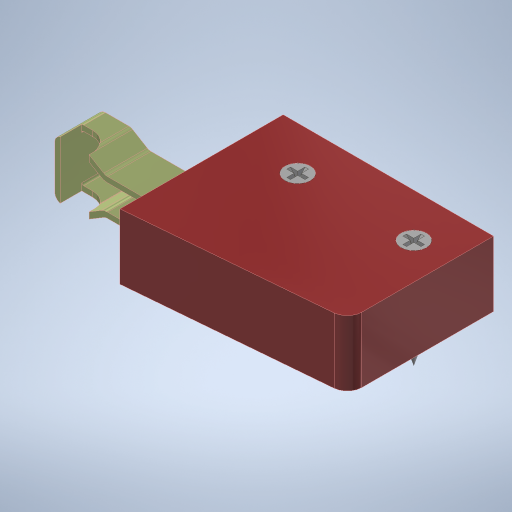
# Autodesk Inventor part: Adjustable universal mounting mechanism T615 Right
Saved by Autodesk Inventor 2024 (Build 280153000, 153)
## iProperties
Category: Wall hanging hardware
Created: 2007-06-13
Part Number: Adjustable universal mounting mechanism T615 Right
Description: Universal adjustable mounting mechanism
Document SubType Name: Modeling
Designer: G.K.
Mass: 44.7999 g
Surface Area: 106.565 cm^2
Volume: 44.7999 cm^3
Density: 1 g/cm^3
Material: Generic
Appearance: Glazed - Firebrick
Authority: Design By CELI APS
Perskaiciuoti: 1
Mase: 0.04479993
Author: G.K.
Title: Universal adjustable mounting mechanism
Subject: Wall hanging hardware
Keywords: Wall hanging hardware, T615, T-600
Comments: Wall hanging hardware, T615, T-600, Wall hanging hardware
Revision Number: 1
Autodesk Inventor part; units mm, degrees
ref_plane "YZ Plane" through (0, 0, 0) normal (1, 0, 0) x (0, 1, 0)
sketch "Sketch1" plane through (0, 0, 0) normal (0, 0, 1) x (1, 0, 0)
  line L0 (0, 0) -> (58, 0)
  line L1 (58, 0) -> (58, -40)
  line L2 (58, -40) -> (0, -45)
  line L3 (0, -45) -> (0, 0)
  dimension "d0" = 45
  dimension "d1" = 58
  dimension "d2" = 40
  constraints: 8 end point, 1 horizontal, 1 parallel, 1 perpendicular
  measures "d0" distance of L2.end L0.start
  measures "d1" distance of L0.start L0.end
  measures "d2" distance of L0.end L1.end
extrude "Extrusion1" add sketch "Sketch1" along normal mid plane 18
ref_plane "Work Plane1" through (0, -23, -9) normal (0, 1, 0) x (1, 0, 0)
sketch "Sketch2" plane through (0, -23, -9) normal (0, 1, 0) x (1, 0, 0)
  line L0 (0, -4) -> (-14, -4)
  line L1 (-14, -4) -> (-14, -14)
  line L2 (-14, -14) -> (0, -14)
  line L3 (0, -14) -> (0, -4)
  line L4 (-19, -1) -> (-28, -1)
  line L5 (-28, -1) -> (-28, -17)
  line L6 (-28, -17) -> (-19, -17)
  line L7 (-19, -17) -> (-19, -1)
  line L8 (-14, -4) -> (-19, -1)
  line L9 (-14, -14) -> (-19, -17)
  line L10 (0, 0) -> (0, -18) projected
  point P0 (0, -9)
  point P1 (0, -9)
  point P2 (-28, -9)
  point P3 (0, -9)
  dimension "d181" = 90
  dimension "d6" = 14
  dimension "d8" = 16
  dimension "d9" = 10
  dimension "d10" = 9
  dimension "d40" = 5
  constraints: 20 end point, 4 midpoint, 4 parallel, 2 horizontal, 2 perpendicular, 1 horizontal alignment
  measures "d6" distance of L0.start L0.end
  measures "d8" distance of L4.end L5.end
  measures "d9" distance between parallel lines of L2 L0
  measures "d10" distance of L4.start L4.end
  measures "d40" horizontal distance of L1.end L6.end
extrude "Extrusion2" add sketch "Sketch2" against normal blind 12
fillet "Fillet1" radius 2 6 edges at (-28, -29, -8) (-28, -29, 8) (-19, -29, -8) (-14, -29, -5) (-14, -29, 5) (-19, -29, 8)
sketch "Sketch5" plane through (0, -23, -9) normal (0, 1, 0) x (1, 0, 0)
  arc A0 (-19.554, -17) -> (-18.525, -16.715) centre (-19.554, -15) ccw projected
  line L0 (-18.525, -16.715) -> (-14.475, -14.285) projected
  arc A1 (-13.446, -14) -> (-14.475, -14.285) centre (-13.446, -16) ccw projected
  line L1 (-13.446, -14) -> (0, -14) projected
  line L2 (0, -4) -> (0, -14) projected
  line L3 (0, -4) -> (-13.446, -4) projected
  arc A2 (-14.475, -3.715) -> (-13.446, -4) centre (-13.446, -2) ccw projected
  line L4 (-14.475, -3.715) -> (-18.525, -1.285) projected
  arc A3 (-18.525, -1.285) -> (-19.554, -1) centre (-19.554, -3) ccw projected
  line L5 (-19.554, -1) -> (-26, -1) projected
  arc A4 (-26, -1) -> (-28, -3) centre (-26, -3) ccw projected
  line L6 (-28, -3) -> (-28, -15) projected
  arc A5 (-28, -15) -> (-26, -17) centre (-26, -15) ccw projected
  line L7 (-26, -17) -> (-19.554, -17) projected
  line L8 (-26, -2.5) -> (-19.554, -2.5)
  arc A6 (-19.2967, -2.5713) -> (-19.554, -2.5) centre (-19.554, -3) ccw
  line L9 (-19.2967, -2.5713) -> (-15.2468, -5.0012)
  arc A7 (-15.2468, -5.0012) -> (-13.446, -5.5) centre (-13.446, -2) ccw
  line L10 (-13.446, -5.5) -> (-1.5, -5.5)
  line L11 (-1.5, -5.5) -> (-1.5, -12.5)
  line L12 (-1.5, -12.5) -> (-13.446, -12.5)
  arc A8 (-13.446, -12.5) -> (-15.2468, -12.9988) centre (-13.446, -16) ccw
  line L13 (-15.2468, -12.9988) -> (-19.2967, -15.4287)
  arc A9 (-19.554, -15.5) -> (-19.2967, -15.4287) centre (-19.554, -15) ccw
  line L14 (-19.554, -15.5) -> (-26, -15.5)
  arc A10 (-26.5, -15) -> (-26, -15.5) centre (-26, -15) ccw
  line L15 (-26.5, -15) -> (-26.5, -3)
  arc A11 (-26, -2.5) -> (-26.5, -3) centre (-26, -3) ccw
  point P0 (0, -9)
  dimension "d18" = 1.5
  constraints: 16 end point, 12 point on circle, 6 centre point, 13 other
  measures "d18" distance between parallel lines of L6 L15
extrude "Extrusion4" cut sketch "Sketch5" against normal through all contours L8 A6 L9 A7 L10 L11 L12 A8 L13 A9 L14 A10 L15 A11
sketch "Sketch4" plane through (0, 0, 0) normal (0, 0, 1) x (1, 0, 0)
  line L0 (-26.5, -23) -> (-26.5, -35) projected
  line L1 (-26.5, -29) -> (-23.5, -29)
  arc A0 (-18.5, -34) -> (-23.5, -29) centre (-23.5, -34) ccw
  line L2 (-18.5, -34) -> (-18.5, -35)
  line L3 (-18.5, -35) -> (-26.5, -35)
  line L4 (-26.5, -35) -> (-26.5, -29)
  line L5 (-26, -23) -> (-19.554, -23) projected
  point P0 (0, 0)
  dimension "d21" = 6
  dimension "d22" = 8
  dimension "d23" = 5
  constraints: 8 end point, 2 perpendicular, 2 point on circle, 2 tangent, 1 centre point, 1 collinear, 1 midpoint, 1 parallel
  measures "d21" distance between parallel lines of L5 L1
  measures "d22" distance of L2.end L0.end
  measures "d23" radius of A0
extrude "Extrusion5" cut sketch "Sketch4" along normal through all both and the other way through all
sketch "Sketch6" plane through (0, 0, 9) normal (0, 0, 1) x (1, 0, 0)
  line L0 (0, 0) -> (58, 0) projected
  line L1 (0, -45) -> (0, 0) projected
  line L2 (16, -12) -> (48, -12)
  dimension "d26" = 12
  dimension "d27" = 32
  dimension "d28" = 16
  constraints: 2 end point, 1 perpendicular
  measures "d26" distance between parallel lines of L0 L2
  measures "d27" distance of L2.end L2.start
  measures "d28" distance from line of L1 L2.start
hole "Hole1" at (16, -12, 9) at (48, -12, 9) direction (0, 0, -1) diameter 5 end through all countersink diameter 7 countersink angle 90
chamfer "Chamfer1" distance 1.5 angle 45 2 edges at (16, -9.5, -9) (48, -9.5, -9)
fillet "Fillet2" radius 4 1 edges at (58, -40, 0)
ref_plane "Work Plane2" through (16, -12, -89.7168) normal (-1, 0, 0) x (0, 0, 1)
sketch "Sketch7" plane through (16, -12, -89.7168) normal (-1, 0, 0) x (0, 0, 1)
  line L0 (98.7168, 3.5) -> (98.7168, -3.5) projected
  line L1 (98.7168, -4.2) -> (98.7168, 0.7) construction
  line L2 (102.1168, 0) -> (68.7168, 0)
  line L3 (98.7168, 0) -> (98.7168, -3.5)
  line L4 (98.7168, -3.5) -> (98.2168, -3.5)
  line L5 (98.2168, -3.5) -> (96.4668, -1.75)
  line L6 (96.4668, -1.75) -> (74.4408, -1.75)
  line L7 (74.4408, -1.75) -> (68.7168, 0)
  point P0 (89.7168, 12)
  point P1 (74.4408, 0)
  dimension "d42" = 3.5
  dimension "d43" = 7
  dimension "d44" = 0.5
  dimension "d45" = 45
  dimension "d46" = 30
  dimension "d47" = 17
  dimension "d48" = 22.026
  constraints: 15 end point, 3 perpendicular, 1 collinear, 1 midpoint, 1 parallel, 1 point on line
  measures "d42" diameter of L6 L2
  measures "d43" diameter of L4 L2
  measures "d44" distance from line of L4.end L3
  measures "d45" angle of L5 L3
  measures "d46" distance from line of L2.end L3
  measures "d47" angle of L7 L2
  measures "d48" distance of L5.end L6.end
revolve "Revolution1" add sketch "Sketch7" angle 360 about axis through (16, -12, 12.4) along (0, 0, -1) separate body
sketch "Sketch8" plane through (16, -12, -89.7168) normal (-1, 0, 0) x (0, 0, 1)
  line L0 (98.7168, 3.5) -> (98.7168, -3.5) projected
  line L1 (96.5568, 0) -> (99.0768, 0)
  line L2 (96.9168, 0) -> (96.9168, 0.9896)
  line L3 (96.9168, 0.9896) -> (98.7168, 2.5)
  line L4 (98.7168, 2.5) -> (98.7168, 0)
  line L5 (98.7168, 3.5) -> (98.7168, -3.5)
  point P0 (89.7168, 12)
  dimension "d50" = 40
  dimension "d51" = 1.8
  dimension "d52" = 2.5
  constraints: 10 end point, 2 perpendicular, 2 point on line, 1 collinear, 1 midpoint
  measures "d50" angle of L3 L1
  measures "d51" distance between parallel lines of L2 L4
  measures "d52" distance from line of L1 L3.end
extrude "Extrusion6" cut sketch "Sketch8" along normal mid plane 1 bodies 2
pattern_circular "Circular Pattern1" count 4 over 360 about axis through (16, -12, -4.263) along (0, 0, -1) of "Extrusion6" bodies 2
thread "Thread1" size "M4x0.7" class "6g" standard "ANSI Metric M Profile" full length
pattern_linear "Rectangular Pattern1" count 2 spacing 32 along (1, 0, 0) bodies 2
sketch "Sketch9" plane through (16, -12, -89.7168) normal (-1, 0, 0) x (0, 0, 1)
  line L0 (80.7168, -3.5) -> (80.7168, 3.5)
  line L1 (80.7168, 4.2) -> (80.7168, -0.7) construction
  line L2 (77.3168, 0) -> (110.7168, 0)
  line L3 (80.7168, 0) -> (80.7168, 3.5)
  line L4 (80.7168, 3.5) -> (81.2168, 3.5)
  line L5 (81.2168, 3.5) -> (82.9668, 1.75)
  line L6 (82.9668, 1.75) -> (104.9928, 1.75)
  line L7 (104.9928, 1.75) -> (110.7168, 0)
  line L8 (80.7168, 4) -> (80.7168, -4) projected
  point P0 (89.7168, 12)
  point P1 (89.7168, 12)
  point P2 (104.9928, 0)
  point P3 (80.7168, 0)
  dimension "d64" = 3.5
  dimension "d65" = 7
  dimension "d66" = 0.5
  dimension "d67" = 45
  dimension "d68" = 30
  dimension "d69" = 17
  dimension "d70" = 22.026
  constraints: 17 end point, 3 perpendicular, 2 midpoint, 1 collinear, 1 parallel, 1 point on line
  measures "d64" diameter of L6 L2
  measures "d65" diameter of L4 L2
  measures "d66" distance from line of L4.end L3
  measures "d67" angle of L5 L3
  measures "d68" distance from line of L2.end L3
  measures "d69" angle of L7 L2
  measures "d70" distance of L5.end L6.end
revolve "Revolution2" [suppressed]
sketch "Sketch10" plane through (16, -12, -89.7168) normal (-1, 0, 0) x (0, 0, 1)
  line L0 (82.8768, 0) -> (80.3568, 0)
  line L1 (82.5168, 0) -> (82.5168, -0.9896)
  line L2 (82.5168, -0.9896) -> (80.7168, -2.5)
  line L3 (80.7168, -2.5) -> (80.7168, 0)
  line L4 (80.7168, -3.5) -> (80.7168, 3.5) projected
  point P0 (89.7168, 12)
  point P1 (80.7168, -3.5)
  point P2 (80.7168, 0)
  point P3 (80.7168, -3.5)
  dimension "d72" = 40
  dimension "d73" = 1.8
  dimension "d74" = 2.5
  constraints: 8 end point, 2 perpendicular, 2 point on line
  measures "d72" angle of L2 L0
  measures "d73" distance between parallel lines of L1 L3
  measures "d74" distance from line of L0 L2.end
extrude "Extrusion7" [suppressed]
pattern_circular "Circular Pattern2" [suppressed]
thread "Thread2" size "M4x0.7" class "6g" standard "ANSI Metric M Profile" full length
pattern_linear "Rectangular Pattern2" [suppressed]
sketch "Sketch11" plane through (0, 0, 0) normal (0, 0, 1) x (1, 0, 0)
  line L0 (-30.5, -54) -> (-30.5, -41)
  arc A0 (-28.5, -39) -> (-30.5, -41) centre (-28.5, -41) ccw
  arc A1 (-28.5, -39) -> (-24.5, -35) centre (-28.5, -35) ccw
  line L1 (-24.5, -35) -> (-24.5, -27)
  line L2 (-24.5, -27) -> (-26.5, -27)
  line L3 (-26.5, -27) -> (-26.5, -35)
  arc A2 (-28.5, -37) -> (-26.5, -35) centre (-28.5, -35) ccw
  arc A3 (-28.5, -37) -> (-32.5, -41) centre (-28.5, -41) ccw
  line L4 (-32.5, -41) -> (-32.5, -54)
  arc A4 (-32.5, -54) -> (-28.5, -58) centre (-28.5, -54) ccw
  line L5 (-28.5, -58) -> (-26.5, -58)
  line L6 (-26.5, -58) -> (-26.5, -56)
  line L7 (-26.5, -56) -> (-28.5, -56)
  arc A5 (-30.5, -54) -> (-28.5, -56) centre (-28.5, -54) ccw
  line L8 (-28, -23) -> (-28, -35) projected
  line L9 (-26, -23) -> (-19.554, -23) projected
  point P0 (0, 0)
  point P1 (-32.5, -37)
  point P2 (-26.5, -27)
  dimension "d86" = 1.5
  dimension "d87" = 4
  constraints: 16 end point, 12 point on circle, 6 centre point
  measures "d86" distance from line of point (-26.5, -27) L8
  measures "d87" distance from line of point (-26.5, -27) L9
extrude "Extrusion8" [suppressed]
sketch "Sketch12" plane through (-24.5, -35, 9) normal (1, 0, 0) x (0, 0, -1)
  line L0 (0, 8) -> (125, 8) projected
  line L1 (125, 8) -> (125, 0) projected
  line L2 (3, 8) -> (122, 8)
  line L3 (122, 8) -> (122, 6)
  line L4 (122, 6) -> (3, 6)
  line L5 (3, 6) -> (3, 8)
  line L6 (0, -23) -> (125, -23) projected
  line L7 (122, 8) -> (120, 6)
  line L8 (3, 8) -> (5, 6)
  point P0 (9, 35)
  point P1 (62.5, 8)
  point P2 (62.5, -23)
  point P3 (62.5, 6)
  dimension "d92" = 2
  dimension "d93" = 3
  dimension "d94" = 2
  dimension "d95" = 2
  constraints: 12 end point, 3 midpoint, 3 point on line, 2 parallel, 2 perpendicular, 2 vertical alignment, 1 horizontal
  measures "d92" distance between parallel lines of L0 L4
  measures "d93" distance between parallel lines of L3 L1
  measures "d94" distance of L7.end L3.end
  measures "d95" distance of L8.end L4.end
extrude "Extrusion9" [suppressed]
sketch "Sketch14" plane through (-30.5, -54, 9) normal (1, 0, 0) x (0, 0, -1)
  line L0 (0, 0) -> (0, 13) projected
  line L1 (125, 13) -> (125, 0) projected
  line L2 (62.5, -3.9613) -> (62.5, 48.6353) construction
  line L3 (0, -4) -> (125, -4) projected
  line L4 (0, 13) -> (0, 0)
  line L5 (49.5, 10.5) -> (39.5, 10.5)
  line L6 (39.5, 2.5) -> (49.5, 2.5)
  arc A0 (39.5, 10.5) -> (39.5, 2.5) centre (39.5, 6.5) ccw
  arc A1 (49.5, 2.5) -> (49.5, 10.5) centre (49.5, 6.5) ccw
  line L7 (35.5, 10.5) -> (53.5, 10.5) construction
  line L8 (53.5, 10.5) -> (53.5, 2.5) construction
  line L9 (53.5, 2.5) -> (35.5, 2.5) construction
  line L10 (35.5, 2.5) -> (35.5, 10.5) construction
  line L11 (62.5, -17.1) -> (62.5, 26.3) construction
  circle A2 centre (28.5, 6.5) radius 3
  line L12 (28.5, 6.5) -> (28.5, 32.5416) construction
  line L13 (21.5, 2.5) -> (21.5, 10.5) construction
  arc A3 (17.5, 2.5) -> (17.5, 10.5) centre (17.5, 6.5) ccw
  line L14 (7.5, 10.5) -> (17.5, 10.5)
  line L15 (3.5, 10.5) -> (3.5, 2.5) construction
  line L16 (21.5, 10.5) -> (3.5, 10.5) construction
  line L17 (3.5, 2.5) -> (21.5, 2.5) construction
  arc A4 (7.5, 10.5) -> (7.5, 2.5) centre (7.5, 6.5) ccw
  line L18 (17.5, 2.5) -> (7.5, 2.5)
  line L19 (71.5, 10.5) -> (71.5, 2.5) construction
  arc A5 (75.5, 10.5) -> (75.5, 2.5) centre (75.5, 6.5) ccw
  line L20 (75.5, 10.5) -> (85.5, 10.5)
  line L21 (85.5, 2.5) -> (75.5, 2.5)
  line L22 (89.5, 10.5) -> (71.5, 10.5) construction
  line L23 (71.5, 2.5) -> (89.5, 2.5) construction
  arc A6 (85.5, 2.5) -> (85.5, 10.5) centre (85.5, 6.5) ccw
  line L24 (89.5, 2.5) -> (89.5, 10.5) construction
  circle A7 centre (96.5, 6.5) radius 3
  line L25 (107.5, 2.5) -> (117.5, 2.5)
  line L26 (117.5, 10.5) -> (107.5, 10.5)
  line L27 (121.5, 2.5) -> (103.5, 2.5) construction
  arc A8 (117.5, 2.5) -> (117.5, 10.5) centre (117.5, 6.5) ccw
  line L28 (103.5, 10.5) -> (121.5, 10.5) construction
  line L29 (103.5, 2.5) -> (103.5, 10.5) construction
  arc A9 (107.5, 10.5) -> (107.5, 2.5) centre (107.5, 6.5) ccw
  line L30 (121.5, 10.5) -> (121.5, 2.5) construction
  point P0 (9, 54)
  point P1 (117.5, 6.5)
  point P2 (62.5, -4)
  point P3 (0, 6.5)
  dimension "d105" = 10.5
  dimension "d106" = 7.5
  dimension "d107" = 18
  dimension "d108" = 8
  dimension "d109" = 18
  dimension "d110" = 6
  dimension "d111" = 7
  dimension "d112" = 7.5
  dimension "d113" = 10.5
  constraints: 56 end point, 32 symmetric about line, 16 point on circle, 10 centre point, 6 tangent, 5 parallel, 2 collinear, 2 horizontal, 2 horizontal alignment, 1 midpoint, 1 perpendicular, 7 other
  measures "d105" distance from line of point (117.5, 6.5) L3
  measures "d106" distance from line of L1 point (117.5, 6.5)
  measures "d107" distance of L7.start L8.start
  measures "d108" distance of L9.end L7.start
  measures "d109" diameter of L8 L11
  measures "d110" diameter of A2
  measures "d111" distance from line of L10 L12.start
  measures "d112" distance from line of point (7.5, 6.5) L0
  measures "d113" distance from line of point (7.5, 6.5) L3
extrude "Extrusion10" [suppressed]
ref_plane "Work Plane4" through (-32.5, -47.5, -19.5) normal (0, 0, -1) x (1, 0, 0)
revolve "Revolution3" [suppressed]
sketch "Sketch16" plane through (-32.5, -47.5, -19.5) normal (0, 0, -1) x (1, 0, 0)
  line L0 (2, 5) -> (2, -5) projected
  line L1 (-0.16, 0) -> (2.36, 0)
  line L2 (0.2, 0) -> (0.2, 2.4896)
  line L3 (0.2, 2.4896) -> (2, 4)
  line L4 (2, 4) -> (2, 0)
  line L5 (2, 5) -> (2, -5)
  point P0 (32.5, -47.5)
  dimension "d125" = 40
  dimension "d126" = 1.8
  dimension "d127" = 4
  constraints: 10 end point, 2 perpendicular, 2 point on line, 1 collinear, 1 midpoint
  measures "d125" angle of L3 L1
  measures "d126" distance between parallel lines of L2 L4
  measures "d127" distance from line of L1 L3.end
extrude "Extrusion11" [suppressed]
pattern_circular "Circular Pattern3" [suppressed]
thread "Thread3" size "M5x0.8" class "6g" standard "ANSI Metric M Profile" length 35
pattern_linear "Rectangular Pattern3" [suppressed]
extrude "Extrusion12" [suppressed]
sketch "Sketch17" plane through (-24.5, -35, 116) normal (1, 0, 0) x (0, 0, -1)
  line L0 (0, 8) -> (125, 8) projected
  line L1 (0, 0) -> (0, 8) projected
  line L2 (125, 8) -> (125, 0) projected
  line L3 (3, 8) -> (122, 8)
  line L4 (122, 8) -> (122, 6)
  line L5 (122, 6) -> (3, 6)
  line L6 (3, 6) -> (3, 8)
  line L7 (122, 8) -> (120, 6)
  line L8 (3, 8) -> (5, 6)
  point P0 (116, 35)
  dimension "d143" = 3
  dimension "d144" = 2
  dimension "d145" = 2
  dimension "d146" = 2
  dimension "d147" = 3
  constraints: 12 end point, 3 point on line, 2 parallel, 2 perpendicular, 1 horizontal
  measures "d143" distance between parallel lines of L4 L2
  measures "d144" distance between parallel lines of L0 L5
  measures "d145" distance from line of L8.end L6
  measures "d146" distance of L4.end L7.end
  measures "d147" distance from line of L5.end L1
extrude "Extrusion13" [suppressed]
sketch "Sketch18" plane through (-30.5, -54, 116) normal (1, 0, 0) x (0, 0, -1)
  line L0 (0, 0) -> (0, 13) projected
  line L1 (0, -4) -> (125, -4) projected
  line L2 (0, 13) -> (0, 0)
  line L3 (49.5, 10.5) -> (39.5, 10.5)
  line L4 (39.5, 2.5) -> (49.5, 2.5)
  arc A0 (39.5, 10.5) -> (39.5, 2.5) centre (39.5, 6.5) ccw
  arc A1 (49.5, 2.5) -> (49.5, 10.5) centre (49.5, 6.5) ccw
  line L5 (35.5, 10.5) -> (53.5, 10.5) construction
  line L6 (53.5, 10.5) -> (53.5, 2.5) construction
  line L7 (53.5, 2.5) -> (35.5, 2.5) construction
  line L8 (35.5, 2.5) -> (35.5, 10.5) construction
  line L9 (62.5, -17.1) -> (62.5, 26.3) construction
  circle A2 centre (28.5, 6.5) radius 3
  line L10 (28.5, 6.5) -> (28.5, 32.5416) construction
  line L11 (21.5, 2.5) -> (21.5, 10.5) construction
  arc A3 (17.5, 2.5) -> (17.5, 10.5) centre (17.5, 6.5) ccw
  line L12 (7.5, 10.5) -> (17.5, 10.5)
  line L13 (3.5, 10.5) -> (3.5, 2.5) construction
  line L14 (21.5, 10.5) -> (3.5, 10.5) construction
  line L15 (3.5, 2.5) -> (21.5, 2.5) construction
  arc A4 (7.5, 10.5) -> (7.5, 2.5) centre (7.5, 6.5) ccw
  line L16 (17.5, 2.5) -> (7.5, 2.5)
  line L17 (89.5, 2.5) -> (89.5, 10.5) construction
  circle A5 centre (96.5, 6.5) radius 3
  line L18 (103.5, 2.5) -> (103.5, 10.5) construction
  arc A6 (107.5, 10.5) -> (107.5, 2.5) centre (107.5, 6.5) ccw
  line L19 (117.5, 10.5) -> (107.5, 10.5)
  line L20 (107.5, 2.5) -> (117.5, 2.5)
  line L21 (103.5, 10.5) -> (121.5, 10.5) construction
  line L22 (121.5, 2.5) -> (103.5, 2.5) construction
  arc A7 (117.5, 2.5) -> (117.5, 10.5) centre (117.5, 6.5) ccw
  line L23 (121.5, 10.5) -> (121.5, 2.5) construction
  line L24 (75.5, 10.5) -> (85.5, 10.5)
  line L25 (85.5, 2.5) -> (75.5, 2.5)
  arc A8 (85.5, 2.5) -> (85.5, 10.5) centre (85.5, 6.5) ccw
  arc A9 (75.5, 10.5) -> (75.5, 2.5) centre (75.5, 6.5) ccw
  line L26 (89.5, 10.5) -> (71.5, 10.5) construction
  line L27 (71.5, 10.5) -> (71.5, 2.5) construction
  line L28 (71.5, 2.5) -> (89.5, 2.5) construction
  point P0 (116, 54)
  point P1 (62.5, -4)
  point P2 (0, 6.5)
  dimension "d150" = 7.5
  dimension "d151" = 10.5
  dimension "d152" = 18
  dimension "d153" = 8
  dimension "d154" = 18
  dimension "d155" = 6
  dimension "d156" = 7
  constraints: 54 end point, 32 symmetric about line, 16 point on circle, 10 centre point, 6 tangent, 4 parallel, 2 collinear, 2 horizontal, 2 horizontal alignment, 1 midpoint, 1 perpendicular, 7 other
  measures "d150" distance from line of point (7.5, 6.5) L0
  measures "d151" distance from line of point (7.5, 6.5) L1
  measures "d152" distance of L8.end L5.end
  measures "d153" distance of L8.start L8.end
  measures "d154" diameter of L6 L9
  measures "d155" diameter of A2
  measures "d156" distance from line of L8 L10.start
extrude "Extrusion14" [suppressed]
ref_plane "Work Plane5" through (-30.5, -47.5, 87.5) normal (0, 0, 1) x (-1, 0, 0)
revolve "Revolution4" [suppressed]
sketch "Sketch21" plane through (-30.5, -47.5, 87.5) normal (0, 0, 1) x (-1, 0, 0)
  line L0 (2.16, 0) -> (-0.36, 0)
  line L1 (1.8, 0) -> (1.8, -2.4896)
  line L2 (1.8, -2.4896) -> (0, -4)
  line L3 (0, -4) -> (0, 0)
  line L4 (0, -5) -> (0, 5)
  line L5 (0, -3) -> (0, 3) projected
  point P0 (-30.5, -47.5)
  point P1 (0, 0)
  dimension "d182" = 40
  dimension "d183" = 1.8
  dimension "d184" = 4
  constraints: 10 end point, 2 perpendicular, 2 point on line, 1 collinear, 1 midpoint
  measures "d182" angle of L2 L0
  measures "d183" distance between parallel lines of L1 L3
  measures "d184" distance from line of L0 L2.end
extrude "Extrusion15" [suppressed]
pattern_circular "Circular Pattern4" [suppressed]
thread "Thread4" size "M5x0.8" class "6g" standard "ANSI Metric M Profile" length 35
pattern_linear "Rectangular Pattern4" [suppressed]
sketch "Sketch15" plane through (-32.5, -47.5, -19.5) normal (0, 0, -1) x (1, 0, 0)
  line L0 (2, -3.9337) -> (2, 0.9663) construction
  line L1 (2, 0) -> (-48, 0)
  line L2 (2, 0) -> (2, -5)
  line L3 (2, -5) -> (1.5, -5)
  line L4 (1.5, -5) -> (-1, -2.5)
  line L5 (-1, -2.5) -> (-39.8229, -2.5)
  line L6 (-39.8229, -2.5) -> (-48, 0)
  line L7 (2, 3) -> (2, -3) projected
  point P0 (32.5, -47.5)
  point P1 (2, 0)
  dimension "d3" = 18
  dimension "d4" = 0
  dimension "d117" = 5
  dimension "d118" = 10
  dimension "d119" = 0.5
  dimension "d120" = 45
  dimension "d121" = 50
  dimension "d122" = 17
  dimension "d123" = 38.8229
  constraints: 16 end point, 2 perpendicular, 1 collinear, 1 midpoint, 1 parallel
  measures "d117" diameter of L5 L1
  measures "d118" diameter of L3 L1
  measures "d119" distance from line of L3.end L2
  measures "d120" angle of L4 L2
  measures "d121" distance from line of L1.end L2
  measures "d122" angle of L6 L1
  measures "d123" distance of L4.end L5.end
sketch "Sketch20" plane through (-30.5, -47.5, 87.5) normal (0, 0, 1) x (-1, 0, 0)
  line L0 (0, 3.9337) -> (0, -0.9663) construction
  line L1 (0, 0) -> (50, 0)
  line L2 (0, 0) -> (0, 5)
  line L3 (0, 5) -> (0.5, 5)
  line L4 (0.5, 5) -> (3, 2.5)
  line L5 (3, 2.5) -> (41.8229, 2.5)
  line L6 (41.8229, 2.5) -> (50, 0)
  line L7 (0, -3) -> (0, 3)
  line L8 (0, -3) -> (0, 3) projected
  point P0 (-30.5, -47.5)
  point P1 (0, 0)
  point P2 (0, 0)
  dimension "d174" = 5
  dimension "d175" = 10
  dimension "d176" = 0.5
  dimension "d177" = 45
  dimension "d178" = 50
  dimension "d179" = 17
  dimension "d180" = 38.8229
  constraints: 18 end point, 2 midpoint, 2 perpendicular, 1 collinear, 1 parallel
  measures "d174" diameter of L5 L1
  measures "d175" diameter of L3 L1
  measures "d176" distance from line of L3.end L2
  measures "d177" angle of L4 L2
  measures "d178" distance from line of L1.end L2
  measures "d179" angle of L6 L1
  measures "d180" distance of L4.end L5.end
